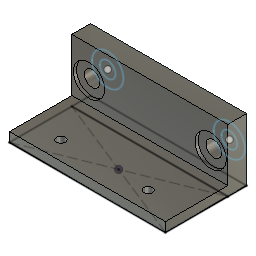
Z Stop Mount (Autodesk Fusion 360 design; units mm, degrees)
Autodesk Fusion 360 part; units mm, degrees
sketch "Sketch1" plane through (0, 0, 0) normal (0, 0, 1) x (1, 0, 0)
  line L0 (25, -10) -> (-25, -10)
  line L1 (-25, -10) -> (-25, 10)
  line L2 (-25, 10) -> (25, 10)
  line L3 (25, 10) -> (25, -10)
  line L4 (25, -10) -> (-25, 10) construction
  line L5 (-25, -10) -> (25, 10) construction
  line L6 (25, 10) -> (-25, 10)
  line L7 (-25, 10) -> (-25, 16)
  line L8 (-25, 16) -> (25, 16)
  line L9 (25, 16) -> (25, 10)
  dimension "d1" = 50
  dimension "d2" = 20
  dimension "d3" = 6
  dimension "d27" = 50
  constraint horizontal L0
  constraint perpendicular L0 L1
  constraint parallel L0 L2
  constraint parallel L1 L3
  constraint coincident L4 origin
  constraint coincident L5 origin
  constraint horizontal L6
  constraint vertical L7
  constraint horizontal L8
  constraint vertical L9
  measures "d1" distance of L1.end L2.end
  measures "d2" distance of L0.end L1.end
  measures "d3" distance of L2.end L8.end
  measures "d27" distance of L7 L9
extrude "Extrude1" add sketch "Sketch1" along normal blind 3 contours L0 L1 L2 L3 L6
extrude "Extrude2" add sketch "Sketch1" along normal blind 20 contours L2 L6 L7 L8 L9
sketch "Sketch2" plane through (0, 16, 0) normal (0, 1, 0) x (-1, 0, 0)
  line L0 (-25, 0) -> (25, 0)
  line L1 (25, 0) -> (25, 20)
  line L2 (25, 20) -> (-25, 20)
  line L3 (-25, 20) -> (-25, 0)
  circle A0 centre (19.5, 10) radius 2.5
  circle A1 centre (-19.5, 10) radius 2.5
  circle A2 centre (-19.5, 10) radius 5
  circle A3 centre (19.5, 10) radius 5
  dimension "d8" = 5
  dimension "d9" = 5
  dimension "d10" = 5.5
  dimension "d11" = 5.5
  dimension "d12" = 10
  dimension "d13" = 10
  constraint concentric A1 A2
  constraint concentric A0 A3
  measures "d8" diameter of A0
  measures "d9" diameter of A1
  measures "d10" distance of L3 A1.centre
  measures "d11" distance of L1 A0.centre
  measures "d12" diameter of A2
  measures "d13" diameter of A3
extrude "Extrude3" cut sketch "Sketch2" against normal up to surface (6 mm away) contours A0 | A1
extrude "Extrude4" cut sketch "Sketch2" along normal blind 1 from surface at -6 contours A2 | A3
sketch "Sketch3" plane through (0, 0, 0) normal (0, 0, -1) x (1, 0, 0)
  line L0 (25, -16) -> (25, 10)
  line L1 (25, 10) -> (-25, 10)
  line L2 (-25, 10) -> (-25, -16)
  line L3 (-25, -16) -> (25, -16)
  circle A0 centre (-14.5, 4) radius 1.4
  circle A1 centre (13.5, 4) radius 1.4
  dimension "d19" = 2.8
  dimension "d20" = 2.8
  dimension "d21" = 28
  dimension "d22" = 6
  dimension "d23" = 6
  dimension "d24" = 10.5
  measures "d19" diameter of A0
  measures "d20" diameter of A1
  measures "d21" horizontal distance of A0.centre A1.centre
  measures "d22" distance of L1 A0.centre
  measures "d23" distance of L1 A1.centre
  measures "d24" distance of L2 A0.centre
extrude "Extrude5" cut sketch "Sketch3" against normal up to surface (3 mm away) contours A0 | A1
equation "d11 = d10"
equation "d23 = d22"
equation "d24 = ( 50 mm - 29 mm ) / 2"
equation "d27 = d1"
